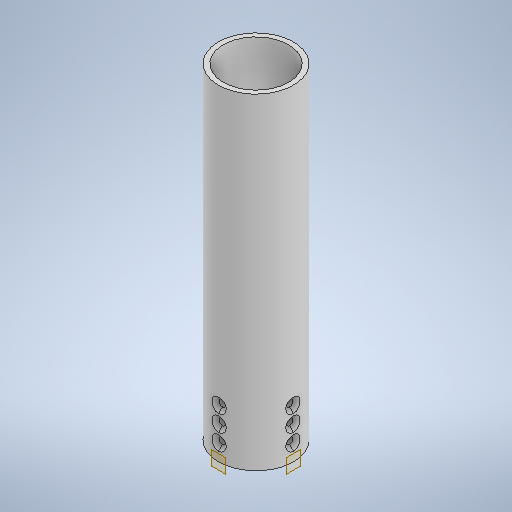
# Autodesk Inventor part: Drifter_Body
Saved by Autodesk Inventor 2025 (Build 290162000, 162)
## iProperties
Created: 2024-05-14
Part Number: Drifter_Body
Material: Generic
Document SubType Name: Modeling
Designer: sml6042
Density: 1 g/cm^3
Appearance: Default
Author: sml6042
Autodesk Inventor part; units mm, degrees
ref_plane "YZ Plane" through (0, 0, 0) normal (1, 0, 0) x (0, 1, 0)
ref_plane "XZ Plane" through (0, 0, 0) normal (0, 1, 0) x (-1, 0, 0)
ref_plane "XY Plane" through (0, 0, 0) normal (0, 0, 1) x (1, 0, 0)
sketch "Sketch1" plane through (0, 0, 0) normal (0, 1, 0) x (-1, 0, 0)
  circle A0 centre (0, 0) radius 57.5
  circle A1 centre (0, 0) radius 50
  dimension "d0" = 115
  dimension "d1" = 100
  constraints: 2 centre point, 2 coincident
  measures "d0" diameter of A0
  measures "d1" diameter of A1
extrude "Extrusion1" add sketch "Sketch1" along normal blind 500 contours A0 | A1
ref_plane "Work Plane5" through (0, 0, 57.5) normal (0, 0, 1) x (1, 0, 0)
sketch "Sketch2" plane through (0, 0, 57.5) normal (0, 0, 1) x (1, 0, 0)
  circle A0 centre (0, 25) radius 5
  line L0 (57.5, 0) -> (-57.5, 0) projected
  circle A1 centre (0, 50) radius 5
  circle A2 centre (0, 75) radius 5
  point P0 (0, 0)
  dimension "d4" = 10
  dimension "d5" = 25
  dimension "d8" = 10
  dimension "d9" = 50
  dimension "d10" = 10
  dimension "d11" = 75
  constraints: 3 centre point
  measures "d4" diameter of A0
  measures "d5" distance of point (0, 0) A0.centre
  measures "d8" diameter of A1
  measures "d9" distance from line of L0 A1.centre
  measures "d10" diameter of A2
  measures "d11" distance from line of L0 A2.centre
extrude "Extrusion2" cut sketch "Sketch2" against normal blind 135
ref_plane "Work Plane3" through (57.5, 0, 0) normal (1, 0, 0) x (0, 1, 0)
sketch "Sketch3" plane through (57.5, 0, 0) normal (1, 0, 0) x (0, 1, 0)
  circle A0 centre (25, 0) radius 5
  circle A1 centre (75, 0) radius 5
  circle A2 centre (50, 0) radius 5
  line L0 (0, -57.5) -> (0, 57.5) projected
  point P0 (0, 0)
  dimension "d14" = 10
  dimension "d15" = 10
  dimension "d16" = 10
  dimension "d17" = 25
  dimension "d18" = 50
  dimension "d19" = 75
  constraints: 3 centre point
  measures "d14" diameter of A0
  measures "d15" diameter of A1
  measures "d16" diameter of A2
  measures "d17" distance from line of L0 A0.centre
  measures "d18" distance from line of L0 A2.centre
  measures "d19" distance from line of L0 A1.centre
extrude "Extrusion3" cut sketch "Sketch3" against normal blind 135
sketch "Sketch4" plane through (0, 500, 0) normal (0, 1, 0) x (1, 0, 0)
  circle A0 centre (0, 0) radius 50
  dimension "d22" = 100
  constraints: 1 centre point, 1 coincident
  measures "d22" diameter of A0
extrude "Extrusion4" cut sketch "Sketch4" against normal blind 340
chamfer "Chamfer1" distance 6 angle 45 4 edges at (3.8236, 71.7782, 57.3727) (-5, 75, 57.2822) (3.8255, 78.2195, 57.3726) (-5, 75.0063, -57.2822)
chamfer "Chamfer2" distance 6 angle 45 20 edges at (3.8236, 46.7782, 57.3727) (-5, 50, 57.2822) (3.8255, 53.2195, 57.3726) (-5, 50.0063, -57.2822) (3.8241, 21.7788, 57.3727) (-5, 25.0028, 57.2822) (3.828, 28.2165, 57.3724) (-4.9999, 25.0341, -57.2822) (-57.2822, 74.9977, -5) (-57.2822, 75.0023, 5) (57.2822, 75.0023, 5) (57.2822, 74.9977, -5) (-57.2822, 49.9977, -5) (-57.2822, 50.0023, 5) (57.2822, 50.0023, 5) (57.2822, 49.9977, -5) (-57.2822, 24.9979, -5) (-57.2822, 25.0021, 5) (57.2822, 25.0021, 5) (57.2822, 24.9979, -5)
body "Solid1"
